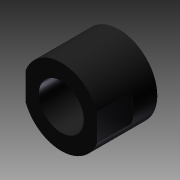
# Autodesk Inventor part: Small Suction Cup Part 3 1764
Saved by Autodesk Inventor 2011 (Build 150239000, 239)
## iProperties
Created: 2011-01-15
Part Number: Small Suction Cup Part 3 1764
Document SubType Name: Modeling
Designer: dfranz
Density: 1 g/cm^3
Author: dfranz
Autodesk Inventor part; units mm, degrees
ref_plane "YZ Plane" through (0, 0, 0) normal (1, 0, 0) x (0, 1, 0)
ref_plane "XZ Plane" through (0, 0, 0) normal (0, 1, 0) x (-1, 0, 0)
ref_plane "XY Plane" through (0, 0, 0) normal (0, 0, 1) x (1, 0, 0)
sketch "Sketch1" plane through (0, 0, 0) normal (0, 0, 1) x (1, 0, 0)
  circle A0 centre (0, 0) radius 9.2075
  circle A1 centre (0, 0) radius 5.3975
  dimension "d0" = 18.415
  dimension "d1" = 10.795
  constraints: 2 centre point, 2 coincident
  measures "d0" diameter of A0
  measures "d1" diameter of A1
extrude "Extrusion1" add sketch "Sketch1" along normal blind 5.6388
sketch "Sketch2" plane through (0, 0, 5.6388) normal (0, 0, 1) x (1, 0, 0)
  circle A0 centre (0, 0) radius 5.3975 projected
  circle A1 centre (0, 0) radius 9.2075 projected
  line L0 (-8.5725, 3.3601) -> (-8.5725, -3.3601)
  line L1 (8.5725, -3.3601) -> (8.5725, 3.3601)
  dimension "d4" = 17.145
  constraints: 4 end point, 4 point on circle, 1 parallel, 1 vertical
  measures "d4" distance between parallel lines of L1 L0
extrude "Extrusion2" add sketch "Sketch2" along normal blind 8.255 contours L1 A1 L0
body "Solid1"
